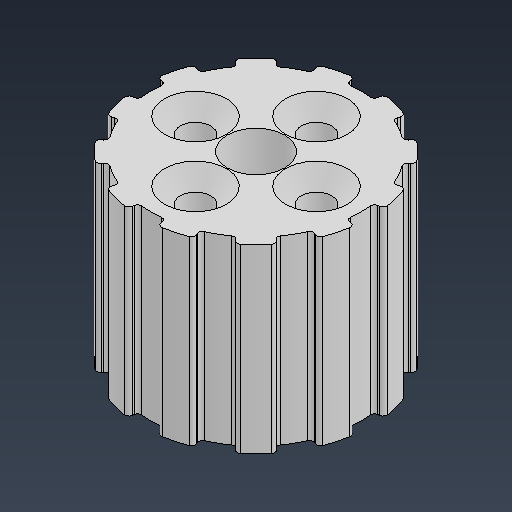
# Autodesk Inventor part: Felga
Saved by Autodesk Inventor 2026.2 (Build 302298010, 298A)
## iProperties
Created: 2026-05-07
Part Number: Felga
Material: Generic
Document SubType Name: Modeling
Designer: szymo
Appearance: Default
Surface Area: 46.033 cm^2
Volume: 3.12448 cm^3
Author: szymo
Autodesk Inventor part; units mm, degrees
ref_plane "YZ Plane" through (0, 0, 0) normal (1, 0, 0) x (0, 1, 0)
ref_plane "XZ Plane" through (0, 0, 0) normal (0, 1, 0) x (-1, 0, 0)
ref_plane "XY Plane" through (0, 0, 0) normal (0, 0, 1) x (1, 0, 0)
sketch "Sketch1" plane through (0, 0, 0) normal (1, 0, 0) x (0, 1, 0)
  line L0 (0, 30) -> (0, -30) construction
  line L1 (0, 5) -> (0.4, 5) construction
  line L2 (0.4, 5) -> (0.4, -5) construction
  line L3 (0.4, -5) -> (0, -5) construction
  line L4 (1, 9.5) -> (9, 9.5) construction
  line L5 (9, 9.5) -> (9, -9.5) construction
  line L6 (9, -9.5) -> (1, -9.5) construction
  line L7 (1, -9.5) -> (1, 9.5) construction
  line L8 (9, -10) -> (0.5, -10)
  line L9 (0.5, -10) -> (0.5, -15)
  line L10 (0.5, -15) -> (19.5, -15) construction
  line L11 (19.5, -15) -> (19.5, -3)
  line L12 (0, 3) -> (19.5, 3) construction
  line L13 (19.5, 3) -> (19.5, -3) construction
  line L14 (19.5, -3) -> (0, -3) construction
  line L15 (9, -10) -> (9, -3)
  line L16 (9, -3) -> (19.5, -3)
  line L17 (0.5, -12) -> (19.5, -12)
  line L18 (3.8567, -6.35) -> (19.5, -6.35) construction
  line L19 (19.5, -3.1) -> (16.25, -6.35) construction
  line L20 (16.25, -6.35) -> (19.5, -9.6) construction
  line L21 (17.75, -4.85) -> (9, -4.85) construction
  line L22 (9, -7.85) -> (17.75, -7.85) construction
  line L23 (0.4, 0) -> (19.5, 0)
  point P0 (0, 0)
  point P1 (0, 0)
  point P2 (13.375, -12)
  point P3 (1, 0)
  dimension "d0" = 30
  dimension "d1" = 30
  dimension "d2" = 5
  dimension "d3" = 5
  dimension "d4" = 0.4
  dimension "d5" = 0.6
  dimension "d6" = 9.5
  dimension "d7" = 9.5
  dimension "d8" = 8
  dimension "d9" = 3
  dimension "d10" = 3
  dimension "d11" = 19.1
  dimension "d13" = 15
  dimension "d14" = 0.1
  dimension "d16" = 3
  dimension "d18" = 0.5
  dimension "d38" = 6
  dimension "d39" = 6.35
  dimension "d40" = 45
  dimension "d41" = 45
  dimension "d42" = 6.5
  dimension "d43" = 1.5
  dimension "d44" = 1.5
  dimension "d45" = 3
  dimension "d93" = 2
  constraints: 48 end point, 16 point on line, 13 perpendicular, 5 midpoint, 3 vertical, 2 horizontal, 2 parallel
  measures "d0" distance of L0.start point (0, 0)
  measures "d1" distance of L0.end point (0, 0)
  measures "d2" distance from line of L1 point (0, 0)
  measures "d3" distance from line of L3 point (0, 0)
  measures "d4" distance between parallel lines of L0 L2
  measures "d5" distance between parallel lines of L2 L7
  measures "d6" vertical distance of point (0, 0) L4.start
  measures "d7" distance from line of L6 point (0, 0)
  measures "d8" distance of L4.start L4.end
  measures "d9" distance from line of L23.start L14
  measures "d10" distance from line of L12 L23.start
  measures "d11" distance between parallel lines of L2 L13
  measures "d13" distance from line of L10 L23.start
  measures "d14" distance between parallel lines of L2 L9
  measures "d16" distance between parallel lines of L10 L17
  measures "d18" distance between parallel lines of L6 L8
  measures "d38" distance between parallel lines of L12 L14
  measures "d39" distance from line of L18 point (1, 0)
  measures "d40" angle of L19 L18
  measures "d41" angle of L18 L20
  measures "d42" distance of L20.end L19.start
  measures "d43" distance between parallel lines of L21 L18
  measures "d44" distance between parallel lines of L22 L18
  measures "d45" distance between parallel lines of L22 L21
  measures "d93" distance between parallel lines of L17 L8
revolve "Revolution2" add sketch "Sketch1" angle 360 about axis through (0, 0.4, 0) along (0, 1, 0)
sketch "Sketch3" plane through (0, 19.5, 0) normal (0, 1, 0) x (1, 0, 0)
  circle A0 centre (0, 0) radius 3 projected
  line L0 (0, 0) -> (-6.35, 0)
  line L1 (0, 0) -> (0, -6.35)
  line L2 (0, 0) -> (6.35, 0)
  line L3 (0, 0) -> (0, 6.35)
  point P0 (0, 0)
  dimension "d59" = 6.35
  dimension "d62" = 360
  constraints: 8 end point, 4 coincident, 1 horizontal, 17 other
  measures "d59" distance of L0.start L0.end
hole "Hole1" at (-6.35, 19.5, 0) at (0, 19.5, 6.35) at (6.35, 19.5, 0) at (0, 19.5, -6.35) direction (0, -1, 0) diameter 3.2 end through all countersink diameter 6.5 countersink angle 90 clearance for "Countersunk Flat Head Screw ISO 2009/7046" size "M3" standard "ISO"
fillet "Fillet1" radius 1 1 edges at (0, 9, 3)
sketch "Sketch5" plane through (0, 0.5, 0) normal (0, -1, 0) x (1, 0, 0)
  circle A0 centre (0, 0) radius 12 projected
  circle A1 centre (0, 0) radius 10 projected
  line L0 (10, 0) -> (12, 0) construction
  circle A2 centre (0, 0) radius 12 projected
  circle A3 centre (0, 0) radius 10 projected
  line L1 (10, 0) -> (0, 0)
  circle A4 centre (0, 0) radius 11
  line L2 (10.9059, 1.4358) -> (11.8973, 1.5663)
  line L3 (10.9059, -1.4358) -> (11.8973, -1.5663)
  line L4 (8.7269, 6.6964) -> (9.5202, 7.3051)
  line L5 (10.1627, 4.2095) -> (11.0866, 4.5922)
  line L6 (4.2095, 10.1627) -> (4.5922, 11.0866)
  line L7 (6.6964, 8.7269) -> (7.3051, 9.5202)
  line L8 (-1.4358, 10.9059) -> (-1.5663, 11.8973)
  line L9 (1.4358, 10.9059) -> (1.5663, 11.8973)
  line L10 (-6.6964, 8.7269) -> (-7.3051, 9.5202)
  line L11 (-4.2095, 10.1627) -> (-4.5922, 11.0866)
  line L12 (-10.1627, 4.2095) -> (-11.0866, 4.5922)
  line L13 (-8.7269, 6.6964) -> (-9.5202, 7.3051)
  line L14 (-10.9059, -1.4358) -> (-11.8973, -1.5663)
  line L15 (-10.9059, 1.4358) -> (-11.8973, 1.5663)
  line L16 (-8.7269, -6.6964) -> (-9.5202, -7.3051)
  line L17 (-10.1627, -4.2095) -> (-11.0866, -4.5922)
  line L18 (-4.2095, -10.1627) -> (-4.5922, -11.0866)
  line L19 (-6.6964, -8.7269) -> (-7.3051, -9.5202)
  line L20 (1.4358, -10.9059) -> (1.5663, -11.8973)
  line L21 (-1.4358, -10.9059) -> (-1.5663, -11.8973)
  line L22 (6.6964, -8.7269) -> (7.3051, -9.5202)
  line L23 (4.2095, -10.1627) -> (4.5922, -11.0866)
  line L24 (10.1627, -4.2095) -> (11.0866, -4.5922)
  line L25 (8.7269, -6.6964) -> (9.5202, -7.3051)
  point P0 (0, 0)
  dimension "d94" = 1
  dimension "d95" = 7.5
  dimension "d96" = 7.5
  dimension "d99" = 360
  constraints: 52 end point, 3 point on circle, 2 horizontal, 2 horizontal alignment, 1 coincident, 81 other
  measures "d95" angle of L2 L0
  measures "d96" angle of L3 L0
extrude "Extrusion4" cut sketch "Sketch5" against normal up to surface (19 mm away) contours A0 L3 A4 L2 | L5 A4 L4 A0 | A0 L25 A4 L24 | L7 A4 L6 A0 | A0 L23 A4 L22 | L9 A4 L8 A0 | A0 L21 A4 L20 | L11 A4 L10 A0 | A0 L19 A4 L18 | L13 A4 L12 A0 | A0 L17 A4 L16 | L15 A4 L14 A0
fillet "Fillet3" radius 0.4 48 edges at (11.0866, 10, 4.5922) (11.8973, 10, 1.5663) (10.9059, 10, 1.4358) (10.1627, 10, 4.2095) (10.9059, 10, -1.4358) (11.8973, 10, -1.5663) (10.1627, 10, -4.2095) (11.0866, 10, -4.5922) (8.7269, 10, -6.6964) (9.5202, 10, -7.3051) (6.6964, 10, -8.7269) (7.3051, 10, -9.5202) (4.2095, 10, -10.1627) (4.5922, 10, -11.0866) (1.4358, 10, -10.9059) (1.5663, 10, -11.8973) (-1.4358, 10, -10.9059) (-1.5663, 10, -11.8973) (-4.2095, 10, -10.1627) (-4.5922, 10, -11.0866) (-6.6964, 10, -8.7269) (-7.3051, 10, -9.5202) (-8.7269, 10, -6.6964) (-9.5202, 10, -7.3051) (-10.1627, 10, -4.2095) (-11.0866, 10, -4.5922) (-10.9059, 10, -1.4358) (-11.8973, 10, -1.5663) (-10.9059, 10, 1.4358) (-11.8973, 10, 1.5663) (-11.0866, 10, 4.5922) (-10.1627, 10, 4.2095) (-8.7269, 10, 6.6964) (-9.5202, 10, 7.3051) (-7.3051, 10, 9.5202) (-6.6964, 10, 8.7269) (-4.2095, 10, 10.1627) (-4.5922, 10, 11.0866) (-1.4358, 10, 10.9059) (-1.5663, 10, 11.8973) (1.4358, 10, 10.9059) (1.5663, 10, 11.8973) (4.2095, 10, 10.1627) (4.5922, 10, 11.0866) (8.7269, 10, 6.6964) (9.5202, 10, 7.3051) (7.3051, 10, 9.5202) (6.6964, 10, 8.7269)
sketch "Sketch6" plane through (0, 19.5, 0) normal (0, 1, 0) x (1, 0, 0)
  point P0 (0, 0)
equation "\"d0\" = d1"
equation "\"d3\" = d2"
equation "\"d7\" = d6"
body "Solid2"
